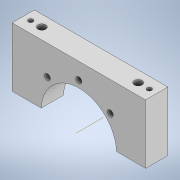
# Autodesk Inventor part: ShooterSeperableClampA
Saved by Autodesk Inventor 2020 (Build 240168000, 168)
## iProperties
Created: 2020-01-29
Part Number: ShooterSeperableClampA
Material: Generic
Document SubType Name: Modeling
Designer: srini
Density: 1 g/cm^3
Appearance: Default
Author: srini
Autodesk Inventor part; units mm, degrees
ref_plane "YZ Plane" through (0, 0, 0) normal (1, 0, 0) x (0, 1, 0)
ref_plane "XZ Plane" through (0, 0, 0) normal (0, 1, 0) x (-1, 0, 0)
ref_plane "XY Plane" through (0, 0, 0) normal (0, 0, 1) x (1, 0, 0)
sketch "Sketch1" plane through (0, 0, 0) normal (0, 0, 1) x (1, 0, 0)
  line L0 (57.15, -25.4) -> (-57.15, -25.4)
  line L1 (-57.15, -25.4) -> (-57.15, 25.4)
  line L2 (-57.15, 25.4) -> (57.15, 25.4)
  line L3 (57.15, 25.4) -> (57.15, -25.4)
  line L4 (57.15, -25.4) -> (-57.15, 25.4) construction
  line L5 (-57.15, -25.4) -> (57.15, 25.4) construction
  point P0 (0, 0)
  point P1 (0, 0)
  point P2 (0, 0)
  dimension "d0" = 114.3
  dimension "d1" = 50.8
  constraints: 12 end point, 3 midpoint, 2 parallel, 1 coincident, 1 horizontal, 1 perpendicular
  measures "d0" distance of L1.end L2.end
  measures "d1" distance of L0.end L1.end
extrude "Extrusion1" add sketch "Sketch1" along normal blind 19.05
sketch "Sketch2" plane through (0, 0, 19.05) normal (0, 0, 1) x (1, 0, 0)
  circle A0 centre (0, -26.67) radius 32.258
  line L0 (-57.15, -25.4) -> (57.15, -25.4) projected
  line L1 (-57.15, 25.4) -> (-57.15, -25.4) projected
  point P0 (0, 0)
  dimension "d4" = 64.516
  dimension "d6" = 1.27
  dimension "d48" = 57.15
  constraints: 1 centre point
  measures "d4" diameter of A0
  measures "d6" distance from line of L0 A0.centre
  measures "d48" distance from line of A0.centre L1
extrude "Extrusion2" cut sketch "Sketch2" against normal through all
sketch "Sketch4" plane through (-57.15, 25.4, 0) normal (0, 1, 0) x (1, 0, 0)
  circle A0 centre (15.875, -9.525) radius 3.3734
  circle A1 centre (98.425, -9.525) radius 3.3734
  line L0 (114.3, 0) -> (0, 0) projected
  line L1 (57.15, -22.86) -> (57.15, 3.81) projected
  dimension "d27" = 6.7469
  dimension "d28" = 9.525
  dimension "d49" = 41.275
  dimension "d50" = 41.275
  constraints: 2 centre point, 1 equal radius, 1 horizontal alignment
  measures "d27" diameter of A0
  measures "d28" distance from line of A0.centre L0
  measures "d49" distance from line of A0.centre L1
  measures "d50" distance from line of A1.centre L1
extrude "Extrusion4" cut sketch "Sketch4" against normal through all
sketch "Sketch5" plane through (-57.15, -25.4, 0) normal (0, -1, 0) x (1, 0, 0)
  circle A0 centre (6.35, 9.525) radius 2.0193
  circle A1 centre (107.95, 9.525) radius 2.0193
  line L0 (0, 0) -> (24.917, 0) projected
  line L1 (57.15, 22.86) -> (57.15, -3.81) projected
  dimension "d33" = 9.525
  dimension "d34" = 4.0386
  dimension "d51" = 50.8
  dimension "d52" = 50.8
  constraints: 2 centre point, 1 equal radius, 1 horizontal alignment
  measures "d33" distance from line of A0.centre L0
  measures "d34" diameter of A0
  measures "d51" distance from line of A0.centre L1
  measures "d52" distance from line of A1.centre L1
extrude "Extrusion5" cut sketch "Sketch5" against normal through all
sketch "Sketch6" plane through (0, 0, 19.05) normal (0, 0, 1) x (1, 0, 0)
  circle A0 centre (-26.9408, 0.2708) radius 2.5797
  arc A1 (32.233, -25.4) -> (-32.233, -25.4) centre (0, -26.67) ccw projected
  circle A2 centre (0, 11.43) radius 2.5797
  circle A3 centre (26.9408, 0.2708) radius 2.5797
  line L0 (0, -26.67) -> (0, -14.487)
  dimension "d39" = 38.1
  dimension "d40" = 5.1594
  dimension "d44" = 90
  dimension "d53" = 45
  constraints: 3 centre point, 2 end point, 1 vertical, 5 other
  measures "d39" distance of A0.centre L0.start
  measures "d40" diameter of A0
extrude "Extrusion6" cut sketch "Sketch6" against normal through all
equation "\"d50\" = d49"
equation "\"d52\" = d51"
body "Solid1"
